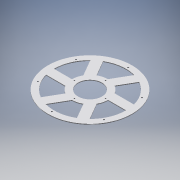
# Autodesk Inventor part: Gear and Turntable Connector
Saved by Autodesk Inventor 2016 (Build 200138000, 138)
## iProperties
Created: 2018-06-21
Part Number: Gear and Turntable Connector
Material: Generic
Document SubType Name: Modeling
Designer: Kade
Density: 1 g/cm^3
Appearance: Aluminum - Dark
Author: Kade
Autodesk Inventor part; units mm, degrees
ref_plane "YZ Plane" through (0, 0, 0) normal (1, 0, 0) x (0, 1, 0)
ref_plane "XZ Plane" through (0, 0, 0) normal (0, 1, 0) x (-1, 0, 0)
ref_plane "XY Plane" through (0, 0, 0) normal (0, 0, 1) x (1, 0, 0)
sketch "Sketch1" plane through (0, 0, 0) normal (0, 1, 0) x (-1, 0, 0)
  circle A0 centre (0, 0) radius 50.8
  circle A1 centre (0, 0) radius 177.8
  line L0 (65.8548, 38.3352) -> (147.4997, 38.3352)
  line L1 (76.1996, 0.2352) -> (152.3998, 0.2352)
  line L2 (-0.2718, 76.1995) -> (40.5506, 146.9061)
  line L3 (37.8962, 66.1084) -> (75.9962, 132.0997)
  line L4 (-66.1266, 37.8643) -> (-106.9491, 108.5709)
  line L5 (-38.3035, 65.8732) -> (-76.4036, 131.8645)
  line L6 (-65.8548, -38.3352) -> (-147.4997, -38.3352)
  line L7 (-76.1996, -0.2352) -> (-152.3998, -0.2352)
  line L8 (0.2718, -76.1995) -> (-40.5506, -146.9061)
  line L9 (-37.8962, -66.1084) -> (-75.9962, -132.0997)
  line L10 (66.1266, -37.8643) -> (106.9491, -108.5709)
  line L11 (38.3035, -65.8732) -> (76.4036, -131.8645)
  arc A2 (66.1266, -37.8643) -> (76.1996, 0.2352) centre (0, 0) ccw
  arc A3 (106.9491, -108.5709) -> (152.3998, 0.2352) centre (0, 0) ccw
  arc A4 (-40.5506, -146.9061) -> (76.4036, -131.8645) centre (0, 0) ccw
  arc A5 (0.2718, -76.1995) -> (38.3035, -65.8732) centre (0, 0) ccw
  arc A6 (-65.8548, -38.3352) -> (-37.8962, -66.1084) centre (0, 0) ccw
  arc A7 (-147.4997, -38.3352) -> (-75.9962, -132.0997) centre (0, 0) ccw
  arc A8 (-106.9491, 108.5709) -> (-152.3998, -0.2352) centre (0, 0) ccw
  arc A9 (-66.1266, 37.8643) -> (-76.1996, -0.2352) centre (0, 0) ccw
  arc A10 (65.8548, 38.3352) -> (37.8962, 66.1084) centre (0, 0) ccw
  arc A11 (-0.2718, 76.1995) -> (-38.3035, 65.8732) centre (0, 0) ccw
  arc A12 (147.4997, 38.3352) -> (75.9962, 132.0997) centre (0, 0) ccw
  arc A13 (40.5506, 146.9061) -> (-76.4036, 131.8645) centre (0, 0) ccw
  dimension "d0" = 101.6
  dimension "d1" = 355.6
  dimension "d4" = 38.1
  dimension "d7" = 360
  dimension "d11" = 25.4
  dimension "d12" = 25.4
  constraints: 24 end point, 24 point on circle, 14 centre point, 4 coincident, 1 horizontal, 1 parallel, 37 other
  measures "d0" diameter of A0
  measures "d1" diameter of A1
  measures "d4" distance between parallel lines of L1 L0
  measures "d11" radial gap between concentric circles of A1 A12
  measures "d12" radial gap between concentric circles of A0 A10
extrude "Extrusion1" add sketch "Sketch1" along normal blind 3.175
sketch "Sketch2" plane through (0, 3.175, 0) normal (0, 1, 0) x (1, 0, 0)
  circle A0 centre (-65.7352, 0) radius 2.5798 projected
  circle A1 centre (0, -65.7352) radius 2.5798 projected
  circle A2 centre (65.7352, 0) radius 2.5798 projected
  circle A3 centre (0, 65.7352) radius 2.5798 projected
  circle A4 centre (-139.741, 80.6795) radius 3.2258 projected
  circle A5 centre (0, 161.3591) radius 3.2258 projected
  circle A6 centre (139.741, 80.6795) radius 3.2258 projected
  circle A7 centre (139.741, -80.6795) radius 3.2258 projected
  circle A8 centre (0, -161.3591) radius 3.2258 projected
  circle A9 centre (-139.741, -80.6795) radius 3.2258 projected
  circle A10 centre (-139.741, 80.6795) radius 3.2258 projected
  point P0 (0, 0)
extrude "Extrusion2" cut sketch "Sketch2" against normal blind 3.175
body "Solid1"
